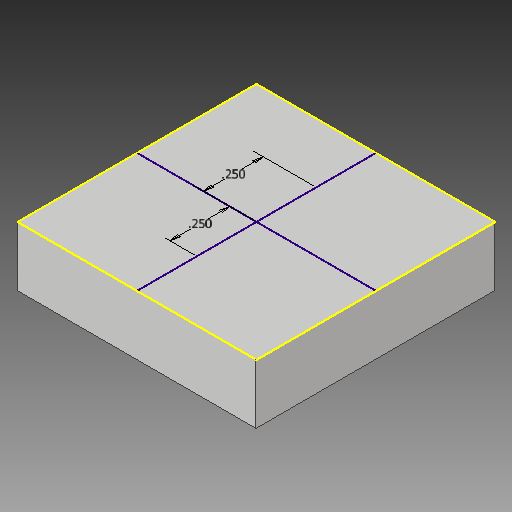
# Autodesk Inventor part: ElectronicsPlateConnector
Saved by Autodesk Inventor 2017 (Build 210142000, 142)
## iProperties
Created: 2018-01-06
Part Number: ElectronicsPlateConnector
Material: Generic
Document SubType Name: Modeling
Designer: User
Density: 1 g/cm^3
Appearance: Default
Author: User
Autodesk Inventor part; units mm, degrees
ref_plane "YZ Plane" through (0, 0, 0) normal (1, 0, 0) x (0, 1, 0)
ref_plane "XZ Plane" through (0, 0, 0) normal (0, 1, 0) x (-1, 0, 0)
ref_plane "XY Plane" through (0, 0, 0) normal (0, 0, 1) x (1, 0, 0)
sketch "Sketch1" plane through (0, 0, 0) normal (0, 0, 1) x (1, 0, 0)
  line L0 (0, 0) -> (25.4, 0)
  line L1 (25.4, 0) -> (25.4, 6.35)
  line L2 (25.4, 6.35) -> (0, 6.35)
  line L3 (0, 6.35) -> (0, 0)
  dimension "d0" = 25.4
  dimension "d1" = 6.35
  constraints: 8 end point, 2 parallel, 1 horizontal, 1 perpendicular
  measures "d0" distance of L2.end L1.end
  measures "d1" distance of L1.end L0.end
extrude "Extrusion1" add sketch "Sketch1" along normal blind 25.4
sketch "Sketch2" plane through (0, 6.35, 0) normal (0, 1, 0) x (1, 0, 0)
  line L0 (0, 0) -> (25.4, 0) projected
  line L1 (12.7, 0) -> (12.7, -25.4)
  line L2 (0, -25.4) -> (25.4, -25.4) projected
  line L3 (0, 0) -> (0, -25.4) projected
  line L4 (0, -12.7) -> (25.4, -12.7)
  line L5 (25.4, 0) -> (25.4, -25.4) projected
  line L6 (12.7, -12.7) -> (12.7, -6.35)
  line L7 (12.7, -12.7) -> (12.7, -19.05)
  dimension "d4" = 6.35
  dimension "d5" = 6.35
  constraints: 8 end point, 5 midpoint, 2 point on line
  measures "d4" distance of L6.start L6.end
  measures "d5" distance of L6.start L7.end
body "Solid1"
